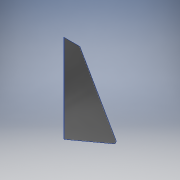
# Autodesk Inventor part: stay_middle
Saved by Autodesk Inventor 2018.1 (Build 221171000, 171)
## iProperties
Created: 2017-10-18
Part Number: stay_middle
Material: アルミニウム 6061
Document SubType Name: Modeling
Designer: kuwano
Density: 2.7 g/cm^3
Appearance: アルミニウム - フラット
Mass: 236.173 g
Surface Area: 610.603 cm^2
Volume: 87.4716 cm^3
Author: kuwano
Autodesk Inventor part; units mm, degrees
ref_plane "YZ Plane" through (0, 0, 0) normal (1, 0, 0) x (0, 1, 0)
ref_plane "XZ Plane" through (0, 0, 0) normal (0, 1, 0) x (-1, 0, 0)
ref_plane "XY Plane" through (0, 0, 0) normal (0, 0, 1) x (1, 0, 0)
sketch "スケッチ1" plane through (0, 0, 0) normal (1, 0, 0) x (0, 1, 0)
  line L0 (-90, 103.923) -> (-90, -196.077)
  line L1 (-90, -196.077) -> (90, -300)
  line L2 (-126, 0) -> (126, 0) projected
  line L3 (0, -380.7846) -> (0, 184.7077) projected
  line L4 (-90, 103.923) -> (-38.1407, 52.0638)
  line L5 (-38.1407, 52.0638) -> (90, -300)
  dimension "d0" = 300
  dimension "d5" = 90
  dimension "d6" = 300
  dimension "d7" = 90
  dimension "d32" = 20
  dimension "d33" = 40
  dimension "d34" = 45
  constraints: 9 end point, 1 vertical
  measures "d0" distance of L0.end L0.start
  measures "d5" distance between parallel lines of L0 L3
  measures "d6" distance from line of L2 L1.end
  measures "d7" distance from line of L3 L1.end
  measures "d32" angle of L0 L5
  measures "d33" angle of L5 L1
  measures "d34" angle of L0 L4
extrude "押し出し1" add sketch "スケッチ1" along normal blind 3 contours L4 L5 L2 L0 | L2 L5 L3 L1 L0 | L3 L5 L1
fillet "フィレット1" radius 5 1 edges at (1.5, 90, -300)
sketch "スケッチ3" plane through (3, 0, 0) normal (1, 0, 0) x (0, 0, -1)
  circle A0 centre (245.7766, 34.0822) radius 2.5
  line L0 (196.077, -90) -> (293.1313, 78.1031) projected
  line L1 (287.0911, 85.3015) -> (-52.0638, -38.1407) projected
  circle A1 centre (205.1793, -6.2342) radius 2.5
  circle A2 centre (174.9758, -22.5483) radius 2.5
  circle A3 centre (89.5158, -22.792) radius 2.5
  line L2 (89.5158, -22.792) -> (174.9758, -22.5483)
  point P0 (0, 0)
  dimension "d36" = 34
  dimension "d37" = 5
  dimension "d38" = 5
  dimension "d40" = 58
  dimension "d41" = 63
  dimension "d42" = 34
  dimension "d43" = 5
  dimension "d44" = 5
  dimension "d45" = 19
  dimension "d46" = 34
  dimension "d47" = 52
  dimension "d51" = 85.46
  constraints: 4 centre point, 2 end point
  measures "d36" distance from line of L1 A0.centre
  measures "d37" diameter of A0
  measures "d38" diameter of A1
  measures "d40" distance from line of L1 A1.centre
  measures "d41" distance from line of L1 L2.end
  measures "d42" distance from line of L2.start L1
  measures "d43" diameter of A2
  measures "d44" diameter of A3
  measures "d45" distance from line of L0 A0.centre
  measures "d46" distance from line of L0 A1.centre
  measures "d47" distance from line of L0 L2.end
  measures "d51" horizontal distance of L2.start L2.end
extrude "押し出し3" cut sketch "スケッチ3" against normal through all
